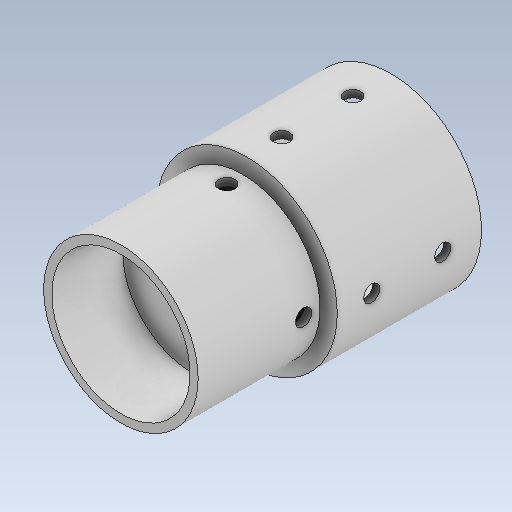
# Autodesk Inventor part: vert_rot
Saved by Autodesk Inventor 2021.4 (Build 254397000, 397)
## iProperties
Created: 2023-11-16
Part Number: vert_rot
Material: Generic
Document SubType Name: Modeling
Designer: vtoth
Density: 1 g/cm^3
Appearance: Default
Author: vtoth
Autodesk Inventor part; units mm, degrees
ref_plane "YZ Plane" through (0, 0, 0) normal (1, 0, 0) x (0, 1, 0)
derived "skeleton_1.ipt"
sketch "Sketch1" plane through (0, 0, 0) normal (0, 1, 0) x (-1, 0, 0)
  line L0 (0, 0) -> (0, 550)
  circle A0 centre (0, 550) radius 6
  line L1 (0, 550) -> (43.8812, 590.9199)
  line L2 (-15.7936, 654.9134) -> (83.0961, 548.8671)
  line L3 (111.4949, 533.0759) -> (80.291, 566.538)
  line L4 (96.8679, 519.4359) -> (65.6639, 552.898)
  line L5 (0, 0) -> (-350, 0)
  line L6 (11.0017, 632.044) -> (5.1509, 626.588)
  point P0 (0, 440)
sketch "Sketch2" plane through (15.7936, 0, 654.9134) normal (-0.6819984, 0, -0.7313537) x (0, -1, 0)
  line L0 (0, -60) -> (0, 0) construction
  line L1 (0, -72) -> (0, 80)
  circle A0 centre (0, 0) radius 10
  line L2 (10, -4.956) -> (10, -4.9245)
  line L3 (-10, 4.9268) -> (-10, 4.959)
  line L4 (-5, 73) -> (5, 73)
  point P0 (0, 0)
  point P1 (0, 0)
  point P2 (0, 0)
  point P3 (0, 10)
  point P4 (0, 10)
  point P5 (0, 10)
  point P6 (0, -57)
  point P7 (0, 45)
sketch "Sketch3" plane through (-42.7147, 0, 709.4732) normal (-0.7313537, 0, 0.6819984) x (0, -1, 0)
  line L0 (0, 0) -> (0, -145) construction
  line L1 (105, 0) -> (-105, 0)
  circle A0 centre (0, 0) radius 6
  line L2 (0, 50) -> (0, -50)
  line L3 (-105, -80) -> (-105, 80)
  point P0 (0, 0)
  point P1 (0, 0)
  point P2 (0, 0)
  point P3 (0, 0)
  point P4 (-79, -23)
ref_plane "Work Plane1" through (15.7936, 0, 654.9134) normal (-0.6819984, 0, -0.7313537) x (0, -1, 0)
ref_plane "Work Plane2" through (-42.7147, 0, 709.4732) normal (-0.7313537, 0, 0.6819984) x (0, -1, 0)
derived "polus.ipt"
sketch "Sketch1_1" plane through (0, 0, 0) normal (0, 1, 0) x (-1, 0, 0)
  line L0 (0, 0) -> (0, 550)
  circle A0 centre (0, 550) radius 6
  line L1 (0, 550) -> (43.8812, 590.9199)
  line L2 (-15.7936, 654.9134) -> (83.0961, 548.8671)
  line L3 (111.4949, 533.0759) -> (80.291, 566.538)
  line L4 (96.8679, 519.4359) -> (65.6639, 552.898)
  line L5 (0, 0) -> (-350, 0)
  line L6 (11.0017, 632.044) -> (5.1509, 626.588)
  point P0 (0, 440)
sketch "Sketch4_1" plane through (0, 0, 0) normal (0, 1, 0) x (-1, 0, 0)
  circle A0 centre (0, 550) radius 6
  line L0 (0, 0) -> (0, 550)
  line L1 (-43, 460) -> (-43, 512)
  line L2 (-43, 512) -> (43, 512)
  line L3 (43, 512) -> (43, 460)
  line L4 (43, 460) -> (39, 460)
  line L5 (39, 460) -> (39, 505)
  line L6 (-39, 505) -> (-39, 460)
  line L7 (-39, 460) -> (-43, 460)
  line L8 (-20, 512) -> (-20, 559.2721)
  line L9 (-20, 559.2721) -> (-7.2721, 572)
  line L10 (-7.2721, 572) -> (7.2721, 572)
  line L11 (7.2721, 572) -> (20, 559.2721)
  line L12 (20, 559.2721) -> (20, 512)
  line L13 (39, 505) -> (0, 505)
  line L14 (0, 512) -> (0, 505)
  line L15 (0, 505) -> (-39, 505)
sketch "Sketch4" plane through (0, 0, 0) normal (0, 1, 0) x (-1, 0, 0)
  line L0 (0, 0) -> (0, 550) projected
  line L1 (-41, 372) -> (-41, 440)
  line L2 (-41, 440) -> (-15.5, 440)
  line L3 (-15.5, 440) -> (-15.5, 443)
  line L4 (-15.5, 443) -> (-27.5, 443)
  line L5 (-27.5, 443) -> (-27.5, 459)
  line L6 (-27.5, 459) -> (-21, 459)
  line L7 (-21, 459) -> (-21, 464)
  line L8 (-21, 464) -> (-30.5, 464)
  line L9 (-30.5, 464) -> (-30.5, 443)
  line L10 (-30.5, 443) -> (-44.5, 443)
  line L11 (-44.5, 443) -> (-44.5, 372)
  line L12 (-44.5, 372) -> (-41, 372)
  line L13 (-34, 445) -> (-38, 445)
  line L14 (-38, 445) -> (-38, 505)
  line L15 (-38, 505) -> (-34, 505)
  line L16 (-34, 505) -> (-34, 470)
  line L17 (-34, 470) -> (-15, 470)
  line L18 (-15, 470) -> (-15, 443)
  line L19 (-15, 443) -> (-27.3, 443)
  line L20 (-27.3, 443) -> (-27.3, 458.8)
  line L21 (-27.3, 458.8) -> (-20, 458.8)
  line L22 (-20, 458.8) -> (-20, 465.5)
  line L23 (-20, 465.5) -> (-34, 465.5)
  line L24 (-34, 465.5) -> (-34, 445)
  line L25 (-20, 470) -> (-20, 465.5)
  line L26 (-15, 465.5) -> (-20, 465.5)
  line L27 (-27.5, 443) -> (-30.5, 443)
  line L28 (0, 505) -> (-39, 505) construction
  point P0 (0, 440)
  dimension "d1" = 82
  dimension "d2" = 3.5
  dimension "d3" = 68
  dimension "d4" = 71
  dimension "d10" = 30
  dimension "d11" = 76
  dimension "d12" = 0
  dimension "d13" = 0.2
  dimension "d14" = 0.2
  dimension "d15" = 1
  dimension "d17" = 3.5
  dimension "dist" = 2
  dimension "d19" = 14
  dimension "d22" = 5
  dimension "d23" = 3
  dimension "d24" = 5
  dimension "d25" = 4.5
  dimension "d26" = 31
  dimension "d27" = 6
  dimension "d51" = 35
  constraints: 54 end point, 22 perpendicular, 4 point on line, 3 parallel, 2 collinear, 1 horizontal
  measures "d1" diameter of L1 L0
  measures "d2" distance between parallel lines of L1 L11
  measures "d3" distance between parallel lines of L2 L12
  measures "d4" distance between parallel lines of L12 L10
  measures "d10" diameter of L18 L0
  measures "d11" diameter of L14 L0
  measures "d12" distance between parallel lines of L4 L19
  measures "d13" distance between parallel lines of L5 L20
  measures "d14" distance between parallel lines of L6 L21
  measures "d15" distance between parallel lines of L7 L22
  measures "d17" distance between parallel lines of L24 L9
  measures "dist" distance between parallel lines of L10 L13
  measures "d19" distance between parallel lines of L11 L9
  measures "d22" distance between parallel lines of L18 L22
  measures "d23" distance between parallel lines of L9 L5
  measures "d24" distance between parallel lines of L8 L6
  measures "d25" distance between parallel lines of L17 L23
  measures "d26" diameter of L3 L0
  measures "d27" distance between parallel lines of L8 L17
  measures "d51" distance between parallel lines of L15 L17
revolve "Revolution1" add sketch "Sketch4" angle 360 about axis through (0, 0, 0) along (0, 0, 1) contours L12 L11 L10 L27 L4 L3 L2 L1 | L9 L8 L7 L6 L5 L27
revolve "Revolution2" add sketch "Sketch4" angle 360 about axis through (0, 0, 0) along (0, 0, 1) separate body contours L4 L20 L21 L22 L26 L18 L19 | L26 L25 L17 L18 | L23 L24 L13 L14 L15 L16 L17 L25
ref_plane "Work Plane3" through (44.5, 0, 443) normal (1, 0, 0) x (0, 1, 0)
sketch "Sketch7" plane through (44.5, 0, 443) normal (1, 0, 0) x (0, 1, 0)
  line L0 (0, 0) -> (0, -71) construction
  line L1 (44.5, -71) -> (-44.5, -71) construction
  circle A0 centre (0, -52) radius 4
  circle A1 centre (0, -17) radius 4
  point P0 (0, -443)
  dimension "d29" = 19
  dimension "d30" = 35
  dimension "d32" = 8
  dimension "d33" = 8
  constraints: 2 centre point, 2 coincident, 2 point on line
  measures "d29" distance from line of L1 point (0, -52)
  measures "d30" distance of point (0, -52) point (0, -17)
  measures "d32" diameter of A0
  measures "d33" diameter of A1
ref_plane "Work Plane4" through (38, 0, 445) normal (1, 0, 0) x (0, 1, 0)
sketch "Sketch8" plane through (38, 0, 445) normal (1, 0, 0) x (0, 1, 0)
  line L0 (0, 0) -> (0, 60) construction
  line L1 (38, 0) -> (-38, 0) construction
  circle A0 centre (0, 8) radius 4
  point P0 (0, -445)
  dimension "d31" = 8
  dimension "d34" = 8
  constraints: 1 centre point, 1 coincident, 1 point on line
  measures "d31" distance from line of L1 point (0, 8)
  measures "d34" diameter of A0
extrude "Extrusion1" cut sketch "Sketch7" against normal up to surface round surface about axis through (0, 0, 406) along (0, 0, 1) radius 41 far side no bodies 1
extrude "Extrusion2" cut sketch "Sketch8" against normal up to surface round surface about axis through (0, 0, 455.25) along (0, 0, 1) radius 34 far side no bodies 2
thread "Thread1" size "M8x1.25" class "6H" standard "ISO Metric profile" length 7
thread "Thread2" size "M8x1.25" class "6H" standard "ANSI Metric M Profile" length 7
thread "Thread3" size "M8x1.25" class "6H" standard "ANSI Metric M Profile" length 7
pattern_circular "Circular Pattern1" count 4 over 360 about axis through (0, 0, 475) along (0, 0, 1) of "Extrusion2" bodies 2
pattern_circular "Circular Pattern2" count 4 over 360 about axis through (0, 0, 407.5) along (0, 0, 1) of "Extrusion1" bodies 1
